Odrive Rack_v1 (Autodesk Fusion 360 design; units mm, degrees)
Autodesk Fusion 360 part; units mm, degrees
sketch "Sketch1" plane through (0, 0, 0) normal (0, 0, 1) x (1, 0, 0)
  line L0 (0, 0) -> (37.5, 0)
  line L1 (37.5, 0) -> (37.5, 30)
  line L2 (0, 0) -> (37.5, 0) construction
  line L3 (37.5, 30) -> (42.5, 30)
  line L4 (42.5, 30) -> (42.5, -40.5)
  line L5 (42.5, -40.5) -> (107.5, -40.5)
  line L6 (107.5, -40.5) -> (107.5, -157.5)
  line L7 (107.5, -157.5) -> (0, -157.5)
  line L8 (0, 0) -> (0, -157.5)
  dimension "d1" = 37.5
  dimension "d2" = 30
  dimension "d3" = 5
  dimension "d4" = 70.5
  dimension "d5" = 65
  dimension "d6" = 117
  dimension "d7" = 107.5
  dimension "d8" = 187.5
  constraint horizontal L0
  constraint vertical L1
  constraint coincident L0.start L2.start
  constraint perpendicular L1 L3
  constraint perpendicular L4 L5
  constraint perpendicular L5 L6
  constraint perpendicular L6 L7
  constraint perpendicular L7 L8
  measures "d1" distance of L0.start L0.end
  measures "d2" distance of L0.end L1.end
  measures "d3" distance of L1.end L3.end
  measures "d4" distance of L3.end L4.end
  measures "d5" distance of L4.end L5.end
  measures "d6" distance of L5.end L6.end
  measures "d7" distance of L6.end L7.end
  measures "d8" distance of L3 L7
extrude "Extrude1" add sketch "Sketch1" along normal blind 5
equation "d1 = ( 75 / 2 ) * 1 mm"
equation "d5 = 20 mm + ( 15 * 3 ) * 1 mm"
equation "d6 = 67 mm + 20 mm + ( 10 * 3 ) * 1 mm"
equation "d7 = d1 + d3 + d5"
